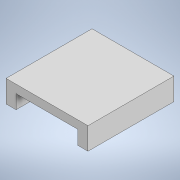
# Autodesk Inventor part: ExpansionCard1
Saved by Autodesk Inventor 2022 (Build 260153000, 153)
## iProperties
Created: 2021-11-01
Part Number: ExpansionCard1
Material: Generic
Document SubType Name: Modeling
Designer: Josh
Density: 1 g/cm^3
Appearance: Default
Author: Josh
Autodesk Inventor part; units mm, degrees
ref_plane "YZ Plane" through (0, 0, 0) normal (1, 0, 0) x (0, 1, 0)
ref_plane "XZ Plane" through (0, 0, 0) normal (0, 1, 0) x (-1, 0, 0)
ref_plane "XY Plane" through (0, 0, 0) normal (0, 0, 1) x (1, 0, 0)
sketch "Sketch1" plane through (38.1, 172.72, 38.1) normal (0, 1, 0) x (-1, 0, 0)
  line L0 (38.1, 773.5975) -> (-850.9, 773.5975)
  line L1 (38.1, 773.5975) -> (165.1, 773.5975)
  line L2 (165.1, 773.5975) -> (165.1, -38.1)
  line L3 (165.1, -38.1) -> (165.1, -241.3)
  line L4 (165.1, -241.3) -> (-850.9, -241.3)
  line L5 (-850.9, -241.3) -> (-850.9, 773.5975)
  line L6 (165.1, -241.3) -> (165.1, -292.1)
  line L7 (165.1, -292.1) -> (-850.9, -292.1)
  line L8 (-850.9, -292.1) -> (-850.9, -241.3)
  point P0 (38.1, -38.1)
  dimension "d0" = 889
  dimension "d1" = 127
  dimension "d2" = 203.2
  dimension "d3" = 1014.8975
  dimension "d4" = 811.6975
  dimension "d9" = 50.8
  constraints: 18 end point, 4 perpendicular, 2 horizontal, 1 point on line, 1 vertical
  measures "d0" distance of L0.start L0.end
  measures "d1" distance of L0.start L1.end
  measures "d2" distance of L2.end L3.end
  measures "d3" distance of L4.end L0.end
  measures "d4" distance of L1.end L2.end
  measures "d9" distance of L3.end L6.end
sketch "Sketch2" plane through (0, 15.24, 0) normal (0, 0, -1) x (-1, 0, 0)
  line L0 (-309.1034, 107.227) -> (-309.1034, 38.647)
  line L1 (-272.9596, 74.2658) -> (-488.8596, 74.2658)
  line L2 (-272.9596, 38.647) -> (-488.8596, 38.647)
  line L3 (-488.8596, 38.647) -> (-488.8596, 107.227)
  line L4 (-488.8596, 107.227) -> (-272.9596, 107.227)
  line L5 (-272.9596, 107.227) -> (-272.9596, 38.647)
  point P0 (0, -15.24)
  dimension "d5" = 215.9
  dimension "d6" = 68.58
  constraints: 12 end point, 2 horizontal, 2 parallel, 1 perpendicular, 1 vertical
  measures "d5" distance of L1.start L1.end
  measures "d6" distance of L0.start L0.end
ref_plane "Work Plane1" through (272.9596, 122.4669, 0) normal (0, 1, 0) x (1, 0, 0)
sketch "Sketch3" plane through (272.9596, 122.4669, 0) normal (0, 1, 0) x (1, 0, 0)
  point P0 (-272.9596, 0)
extrude "Extrusion2" add sketch "Sketch1" along normal blind 101.6
sketch "Sketch4" plane through (38.1, 172.72, 38.1) normal (0, -1, 0) x (1, 0, 0)
  line L0 (-165.1, -292.1) -> (-165.1, 773.5975) projected
  line L1 (-165.1, -292.1) -> (-165.1, 773.5975)
  line L2 (-165.1, 773.5975) -> (-38.1, 773.5975)
  line L3 (-165.1, 773.5975) -> (850.9, 773.5975) projected
  line L4 (-38.1, -38.1) -> (-38.1, 773.5975)
  line L5 (-38.1, -38.1) -> (723.083, -38.1)
  line L6 (723.083, -38.1) -> (723.083, 773.5975)
  line L7 (723.083, 773.5975) -> (850.9, 773.5975)
  line L8 (850.9, 773.5975) -> (850.9, -292.1) projected
  line L9 (850.9, 773.5975) -> (850.9, -292.1)
  line L10 (850.9, -292.1) -> (-165.1, -292.1) projected
  line L11 (850.9, -292.1) -> (-165.1, -292.1)
  constraints: 16 end point, 3 perpendicular, 3 point on line, 2 collinear, 1 horizontal
extrude "Extrusion3" add sketch "Sketch4" along normal blind 172.72 contours L0 L2 L4 L5 L6 L3 L8 L10
extrude "Extrusion4" cut sketch "Sketch2" along normal blind 203.2
sketch "Sketch5" plane through (761.183, 172.72, 0) normal (-1, 0, 0) x (0, 0, 1)
  line L0 (0, -172.72) -> (811.6975, -172.72) projected
  line L1 (0, 0) -> (0, -172.72) projected
  line L2 (811.6975, -172.72) -> (0, -172.72)
  line L3 (0, -172.72) -> (0, 0)
  line L4 (0, 0) -> (811.6975, 0)
  line L5 (811.6975, 0) -> (811.6975, -172.72)
  point P0 (0, -172.72)
  constraints: 8 end point, 2 parallel, 1 horizontal, 1 perpendicular
extrude "Extrusion5" cut sketch "Sketch5" against normal blind 2.54
sketch "Sketch6" plane through (0, 172.72, 811.6975) normal (1, 0, 0) x (0, 0, -1)
  line L0 (0, -172.72) -> (1065.6975, -172.72) projected
  line L1 (0, 0) -> (811.6975, 0) projected
  line L2 (0, -172.72) -> (811.6975, -172.72)
  line L3 (811.6975, -172.72) -> (811.6975, 0)
  line L4 (811.6975, 0) -> (0, 0)
  line L5 (0, 0) -> (0, -172.72)
  point P0 (811.6975, -172.72)
  constraints: 8 end point, 2 parallel, 1 horizontal, 1 perpendicular
extrude "Extrusion6" cut sketch "Sketch6" against normal blind 2.54
body "Solid1"
